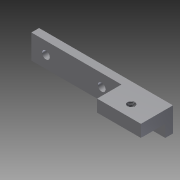
# Autodesk Inventor part: alpha_omega_holder
Saved by Autodesk Inventor 2011 (Build 150239000, 239)
## iProperties
Created: 2011-03-31
Part Number: alpha_omega_holder
Document SubType Name: Modeling
Designer: labuser
Density: 1 g/cm^3
Author: labuser
Autodesk Inventor part; units mm, degrees
ref_plane "YZ Plane" through (0, 0, 0) normal (1, 0, 0) x (0, 1, 0)
ref_plane "XZ Plane" through (0, 0, 0) normal (0, 1, 0) x (-1, 0, 0)
ref_plane "XY Plane" through (0, 0, 0) normal (0, 0, 1) x (1, 0, 0)
sketch "Sketch1" plane through (0, 0, 0) normal (0, 0, 1) x (1, 0, 0)
  line L0 (0, 0) -> (55, 0)
  line L1 (55, 0) -> (55, 10)
  line L2 (55, 10) -> (0, 10)
  line L3 (0, 10) -> (0, 0)
  dimension "d0" = 55
  dimension "d1" = 10
  constraints: 8 end point, 2 parallel, 1 horizontal, 1 perpendicular
  measures "d0" distance of L2.end L1.end
  measures "d1" distance of L1.end L0.end
extrude "Extrusion1" add sketch "Sketch1" along normal blind 3.175
sketch "Sketch3" plane through (0, 0, 3.175) normal (0, 0, 1) x (1, 0, 0)
  line L0 (37, 5) -> (55, 5) projected
  line L1 (0, 10) -> (55, 10) projected
  line L2 (0, 0) -> (6, 0) construction
  line L3 (6, 0) -> (6, 10) construction
  line L4 (6, 10) -> (0, 10) construction
  line L5 (0, 10) -> (0, 0) construction
  line L6 (-4.3576, 5) -> (33.1549, 5) construction
  line L7 (6, 0) -> (28.9, 0) construction
  line L8 (28.9, 0) -> (28.9, 6.8677) construction
  line L9 (28.9, 6.8677) -> (6, 6.8677) construction
  line L10 (6, 6.8677) -> (6, 0) construction
  point P0 (6, 5)
  point P1 (28.9, 5)
  dimension "d8" = 6
  dimension "d9" = 22.9
  constraints: 18 end point, 6 point on line, 4 parallel, 2 horizontal, 2 perpendicular
  measures "d8" distance of L4.end L3.end
  measures "d9" distance of L9.end L8.end
hole "Hole1" at (6, 5, 3.175) at (28.9, 5, 3.175) direction (0, 0, -1) diameter 3.2 end through all
sketch "Sketch6" plane through (0, 0, 3.175) normal (0, 0, 1) x (1, 0, 0)
  line L0 (55, 10) -> (37, 10)
  line L1 (37, 10) -> (37, 5)
  line L2 (37, 5) -> (55, 5)
  line L3 (55, 5) -> (55, 10)
  dimension "d32" = 18
  dimension "d33" = 5
  constraints: 8 end point, 2 parallel, 1 horizontal, 1 perpendicular
  measures "d32" distance of L2.end L1.end
  measures "d33" distance of L1.end L0.end
extrude "Extrusion4" add sketch "Sketch6" along normal blind 10
sketch "Sketch7" plane through (37, 5, 3.175) normal (0, -1, 0) x (1, 0, 0)
  line L0 (18, 0) -> (18, 10) projected
  line L1 (9, 13.1417) -> (9, -6.2593) construction
  line L2 (-2.325, 5) -> (23.2178, 5) construction
  point P0 (-37, -3.175)
  point P1 (9, 5)
  constraints: 4 end point, 2 point on line, 1 parallel, 1 perpendicular
hole "Hole3" at (46, 5, 8.175) direction (0, 1, 0) diameter 3 end through all
thread "Thread2" size "M3x0.5" class "6H" standard "ISO Metric profile" full length
sketch "Sketch8" plane through (55, 0, 0) normal (1, 0, 0) x (0, 0, -1)
  line L0 (-3.175, 5) -> (-13.175, 5) projected
  line L1 (-13.175, 5) -> (-12.775, 5) construction
  line L2 (-12.775, 5) -> (-12.775, 5.2) construction
  line L3 (-12.775, 5.2) -> (-13.175, 5.2) construction
  line L4 (-13.175, 5.2) -> (-13.175, 5) construction
  line L5 (-12.775, 5.2) -> (-12.575, 5)
  line L6 (-12.775, 5.2) -> (-12.4922, 5.2) construction
  line L7 (-12.775, 5.2) -> (-12.975, 5)
  line L8 (-12.775, 5.2) -> (-12.4922, 5.2) construction
  line L9 (-12.975, 5) -> (-12.575, 5)
  dimension "d45" = 0.4
  dimension "d46" = 0.2
  dimension "d47" = 45
  dimension "d48" = 135
  constraints: 18 end point, 3 horizontal, 2 equal length, 2 parallel, 1 collinear, 1 midpoint, 1 perpendicular, 1 point on line
  measures "d45" distance of L3.end L2.end
  measures "d46" distance of L2.end L1.end
  measures "d47" angle of L5 L6
  measures "d48" angle of L7 L8
extrude "Extrusion5" cut sketch "Sketch8" against normal through all
body "Solid1"
